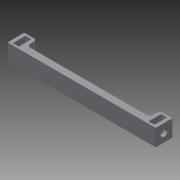
# Autodesk Inventor part: BaseSlat
Saved by Autodesk Inventor 2014 SP1 (Build 180222100, 222)
## iProperties
Created: 2017-05-20
Part Number: BaseSlat
Material: Generic
Document SubType Name: Modeling
Designer: danielsikar
Density: 1 g/cm^3
Appearance: Default
Author: danielsikar
Autodesk Inventor part; units mm, degrees
ref_plane "YZ Plane" through (0, 0, 0) normal (1, 0, 0) x (0, 1, 0)
ref_plane "XZ Plane" through (0, 0, 0) normal (0, 1, 0) x (-1, 0, 0)
sketch "Sketch11" plane through (0, 0, 0) normal (1, 0, 0) x (0, 1, 0)
  line L0 (0, 0) -> (10, 0)
  line L1 (10, 0) -> (10, 10)
  line L2 (10, 10) -> (0, 10)
  line L3 (0, 10) -> (0, 0)
  dimension "d27" = 10
  dimension "d28" = 10
  constraints: 8 end point, 2 parallel, 1 horizontal, 1 perpendicular
  measures "d27" distance of L2.end L1.end
  measures "d28" distance of L1.end L0.end
extrude "Extrusion8" add sketch "Sketch11" along normal blind 88.2
sketch "Sketch12" plane through (0, 0, 0) normal (-1, 0, 0) x (0, 0, 1)
  circle A0 centre (5, 5) radius 2.1
  dimension "d31" = 4.2
  constraints: 1 centre point
  measures "d31" diameter of A0
extrude "Extrusion9" cut sketch "Sketch12" against normal blind 88.2
sketch "Sketch13" plane through (0, 0, 10) normal (0, 0, 1) x (1, 0, 0)
  line L0 (0, 10) -> (0, 0) projected
  line L1 (0, 10) -> (88.2, 10) projected
  line L2 (10, 10) -> (78.2, 10)
  line L3 (78.2, 10) -> (78.2, 4)
  line L4 (78.2, 4) -> (10, 4)
  line L5 (10, 4) -> (10, 10)
  dimension "d34" = 68.2
  dimension "d35" = 6
  dimension "d36" = 10
  constraints: 8 end point, 2 parallel, 1 horizontal, 1 perpendicular, 1 point on line
  measures "d34" distance of L3.end L4.end
  measures "d35" distance of L2.end L3.end
  measures "d36" distance between parallel lines of L5 L0
extrude "Extrusion10" cut sketch "Sketch13" against normal blind 88.2
sketch "Sketch14" plane through (0, 0, 10) normal (0, 0, 1) x (1, 0, 0)
  line L0 (0, 10) -> (10, 10) projected
  line L1 (0, 10) -> (0, 0) projected
  line L2 (2, 8.75) -> (5.5, 8.75)
  line L3 (5.5, 8.75) -> (5.5, 1.25)
  line L4 (5.5, 1.25) -> (2, 1.25)
  line L5 (2, 1.25) -> (2, 8.75)
  line L6 (10, 10) -> (7.5, 10)
  line L7 (7.5, 10) -> (7.5, 4)
  line L8 (7.5, 4) -> (10, 4)
  line L9 (10, 4) -> (10, 10)
  dimension "d39" = 3.5
  dimension "d40" = 7.5
  dimension "d41" = 1.25
  dimension "d42" = 2
  dimension "d43" = 2
  constraints: 16 end point, 4 parallel, 2 horizontal, 2 perpendicular
  measures "d39" distance of L3.end L4.end
  measures "d40" distance of L2.end L3.end
  measures "d41" distance between parallel lines of L2 L0
  measures "d42" distance between parallel lines of L5 L1
  measures "d43" distance between parallel lines of L7 L3
extrude "Extrusion11" cut sketch "Sketch14" against normal blind 88.2
ref_plane "Work Plane5" through (44.1, 0, 0) normal (1, 0, 0) x (0, 0, -1)
mirror "Mirror4" about plane through (44.1, 0, 0) normal (1, 0, 0) of "Extrusion11", "Extrusion10"
sketch "Sketch15" plane through (7.5, 4, 3.1534) normal (0, 1, 0) x (1, 0, 0)
  line L0 (0, 0) -> (0, 3.1534) projected
  line L1 (4, 1.5767) -> (69.2, 1.5767)
  line L2 (69.2, 1.5767) -> (69.2, -5.2793)
  line L3 (69.2, -5.2793) -> (4, -5.2793)
  line L4 (4, -5.2793) -> (4, 1.5767)
  point P0 (-7.5, 3.1534)
  dimension "d47" = 65.2
  dimension "d48" = 4
  constraints: 8 end point, 2 parallel, 1 horizontal, 1 perpendicular
  measures "d47" distance of L2.end L3.end
  measures "d48" distance between parallel lines of L4 L0
extrude "Extrusion12" add sketch "Sketch15" against normal blind 3
fillet "Fillet2" radius 2 6 edges at (80.7, 10, 5) (80.7, 4, 8.4233) (80.7, 4, 1.5767) (7.5, 4, 1.5767) (7.5, 4, 8.4233) (7.5, 10, 5)
body "Solid2"
